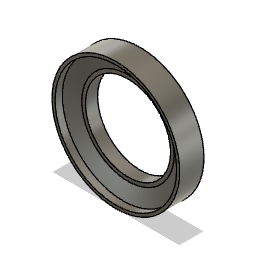
put_robot v1 (Autodesk Fusion 360 design; units mm, degrees)
Autodesk Fusion 360 part; units mm, degrees
sketch "スケッチ1" plane through (0, 0, 0) normal (0, 0, 1) x (1, 0, 0)
  circle A0 centre (0, 0) radius 52.5
  circle A1 centre (0, 0) radius 50
  dimension "d1" = 105
  dimension "d2" = 100
  constraint coincident A0.centre A1.centre
  measures "d1" diameter of A0
  measures "d2" diameter of A1
extrude "押し出し1" add sketch "スケッチ1" along normal blind 7 makes body 1
sketch "スケッチ2" plane through (0, 0, 0) normal (0, 0, 1) x (1, 0, 0)
  circle A0 centre (0, 0) radius 52.5
  circle A1 centre (0, 0) radius 35
  dimension "d5" = 105
  dimension "d6" = 70
  constraint coincident A0.centre A1.centre
  measures "d5" diameter of A0
  measures "d6" diameter of A1
extrude "押し出し2" add sketch "スケッチ2" against normal blind 15 bodies 1
extrude "押し出し3" add 1 faces at (51.2851, -5.0923, 7) along direction (0, 0, 1) blind 2 on bodies 1 bodies 1
extrude "押し出し4" add 1 faces at (51.2851, -5.0923, 9) along direction (0, 0, 1) blind 1 on bodies 1 bodies 1
extrude "押し出し5" cut 1 faces at (46.4712, -2.6082, -15) along direction (0, 0, 1) blind 5 on bodies 1 bodies 1
sketch "スケッチ3" plane through (0, 0, 0) normal (0, 1, 0) x (1, 0, 0)
  line L0 (50, 0) -> (38.0019, 0)
  line L1 (50, -4) -> (50, 0)
  line L2 (50, -4) -> (38.0019, 0)
  dimension "d16" = 4
  constraint horizontal L0
  constraint vertical L1
  measures "d16" distance of L0.start L1.start
revolve "回転1" add sketch "スケッチ3" angle 360 about axis through (0, 0, 1.75) along (0, 0, 1) separate body makes body 2
